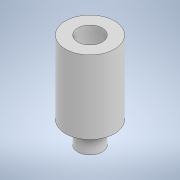
# Autodesk Inventor part: Rodillo2
Saved by Autodesk Inventor 2021 (Build 250183000, 183)
## iProperties
Created: 2021-06-07
Part Number: Rodillo2
Material: Genérico
Document SubType Name: Modeling
Designer: Mecatronica
Density: 1 g/cm^3
Appearance: Valor por defecto
Author: Mecatronica
Autodesk Inventor part; units mm, degrees
ref_plane "YZ Plane" through (0, 0, 0) normal (1, 0, 0) x (0, 1, 0)
ref_plane "XZ Plane" through (0, 0, 0) normal (0, 1, 0) x (-1, 0, 0)
ref_plane "XY Plane" through (0, 0, 0) normal (0, 0, 1) x (1, 0, 0)
sketch "Boceto1" plane through (0, 0, 0) normal (0, 1, 0) x (-1, 0, 0)
  circle A0 centre (0, 0) radius 33.3333
  circle A1 centre (0, 0) radius 16.6667
  dimension "d0" = 66.6667
  dimension "d1" = 33.3333
  constraints: 2 centre point, 2 coincident
  measures "d0" diameter of A0
  measures "d1" diameter of A1
extrude "Extrusión1" add sketch "Boceto1" along normal blind 100
sketch "Boceto2" plane through (0, 0, 0) normal (0, -1, 0) x (1, 0, 0)
  circle A0 centre (0, 0) radius 16.6667 projected
extrude "Extrusión2" add sketch "Boceto2" along normal blind 30
